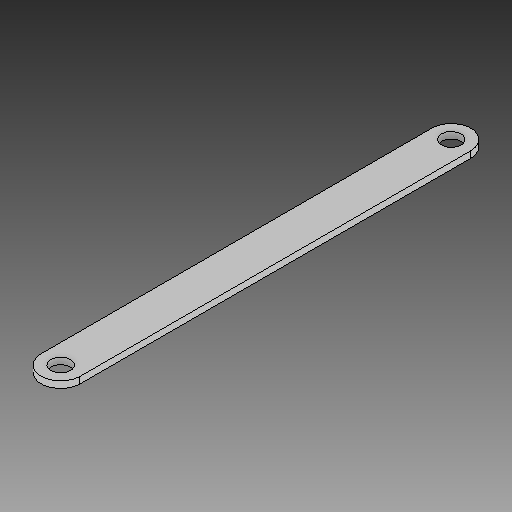
# Autodesk Inventor part: pleuel
Saved by Autodesk Inventor 2018 (Build 220112000, 112)
## iProperties
Created: 2024-05-02
Part Number: pleuel
Material: Generic
Document SubType Name: Modeling
Designer: neo
Density: 1 g/cm^3
Appearance: Default
Mass: 0.373989 g
Surface Area: 9.05677 cm^2
Volume: 0.373989 cm^3
Author: neo
Autodesk Inventor part; units mm, degrees
ref_plane "YZ Plane" through (0, 0, 0) normal (1, 0, 0) x (0, 1, 0)
ref_plane "XZ Plane" through (0, 0, 0) normal (0, 1, 0) x (-1, 0, 0)
ref_plane "XY Plane" through (0, 0, 0) normal (0, 0, 1) x (1, 0, 0)
sketch "Sketch1" plane through (0, 0, 0) normal (0, 1, 0) x (-1, 0, 0)
  line L0 (3.1097, 37.1226) -> (3.1091, -22.999)
  line L1 (9.1067, -23.1206) -> (9.1073, 37.001)
  arc A0 (9.1073, 37.001) -> (3.1097, 37.1226) centre (6.1073, 37.001) ccw
  arc A1 (3.1091, -22.999) -> (9.1067, -23.1206) centre (6.1091, -22.999) ccw
  circle A2 centre (6.1073, 37.001) radius 1.5
  circle A3 centre (6.1091, -22.999) radius 1.5
  point P0 (0, 0)
  dimension "d" = 3
  dimension "d1" = 3
  dimension "d2" = 3
  dimension "d3" = 3
  dimension "d4" = 60
  constraints: 4 centre point, 4 end point, 4 point on circle, 2 coincident, 1 parallel
  measures "d" diameter of A3
  measures "d1" diameter of A2
  measures "d2" radius of A0
  measures "d3" radius of A1
  measures "d4" distance of A0.centre A1.centre
extrude "Extrusion1" add sketch "Sketch1" along normal blind 1
equation "\"d1\" = d"
equation "\"d2\" = d"
equation "\"d3\" = d"
body "Solid1"
